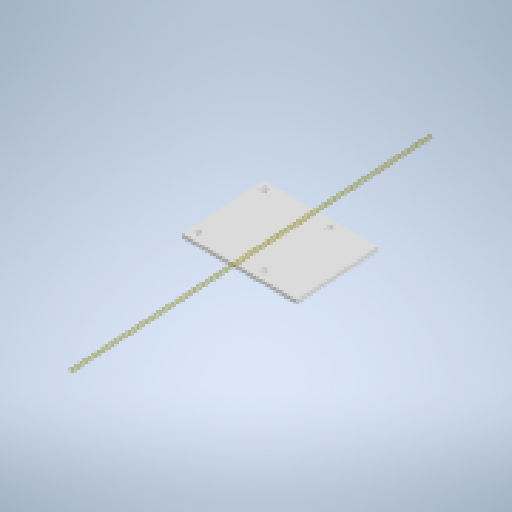
# Autodesk Inventor part: X axis carriage
Saved by Autodesk Inventor 2023.2 (Build 272271000, 271)
## iProperties
Created: 2023-05-09
Part Number: X axis carriage
Material: Generic
Document SubType Name: Modeling
Designer: dmargari
Density: 1 g/cm^3
Appearance: Default
Author: dmargari
Autodesk Inventor part; units mm, degrees
ref_plane "YZ Plane" through (0, 0, 0) normal (1, 0, 0) x (0, 1, 0)
ref_plane "XZ Plane" through (0, 0, 0) normal (0, 1, 0) x (-1, 0, 0)
ref_plane "XY Plane" through (0, 0, 0) normal (0, 0, 1) x (1, 0, 0)
ref_plane "Work Plane1" through (-11.5353, 732.2171, -211.5196) normal (-0.0000012, -0.9978756, -0.0651475) x (1, -0.0000012, -0.0000001)
sketch "Sketch2" plane through (-11.5353, 732.2171, -211.5196) normal (-0.0000012, -0.9978756, -0.0651475) x (1, -0.0000012, -0.0000001)
  line L0 (47.2205, 275.3712) -> (-77.9795, 275.3712)
  line L1 (-77.9795, 275.3712) -> (-77.9795, 150.1712)
  line L2 (-77.9795, 150.1712) -> (47.2205, 150.1712)
  line L3 (47.2205, 150.1712) -> (47.2205, 275.3712) construction
  line L4 (47.2205, 275.3712) -> (97.2205, 275.3712)
  line L5 (97.2205, 275.3712) -> (97.2205, 150.1712)
  line L6 (97.2205, 150.1712) -> (47.2205, 150.1712)
  line L7 (34.9205, 141.5153) -> (34.9205, 309.2543) construction
  line L8 (-65.6795, 309.2543) -> (-65.6795, 110.7061) construction
  line L9 (72.2205, 263.0712) -> (-113.8811, 263.0712) construction
  line L10 (72.2205, 162.4712) -> (-118.8511, 162.4712) construction
  point P0 (11.5362, 258.7723)
  point P1 (-138.0714, 537.573)
  point P2 (-211.9698, 678.1667)
  point P3 (34.9205, 263.0712)
  point P4 (34.9205, 162.4712)
  point P5 (-65.6795, 162.4712)
  point P6 (-65.6795, 263.0712)
  dimension "d15" = 125.2
  dimension "d16" = 125.2
  dimension "d23" = 50
  dimension "d30" = 12.3
  dimension "d31" = 100.6
  dimension "d32" = 12.3
  dimension "d33" = 100.6
  constraints: 22 end point, 9 point on line, 4 perpendicular, 3 horizontal, 2 parallel, 1 collinear, 1 vertical
  measures "d15" distance of L2.end L1.end
  measures "d16" distance of L1.end L0.end
  measures "d23" distance of L0.start L4.end
  measures "d30" distance between parallel lines of L0 L9
  measures "d31" distance between parallel lines of L9 L10
  measures "d32" distance between parallel lines of L3 L7
  measures "d33" distance between parallel lines of L7 L8
extrude "Extrusion2" add sketch "Sketch2" along normal blind 6
hole "Hole1" at (23.3852, 715.0787, 50.9927) at (23.3852, 721.6325, -49.3936) at (-77.2148, 715.0788, 50.9927) direction (-0.0000012, -0.9978756, -0.0651475) diameter 5.1 end through all counterbore diameter 9.2 counterbore depth 2
hole "Hole2" at (-77.2148, 721.6326, -49.3935) direction (-0.0000012, -0.9978756, -0.0651475) diameter 7.2 end through all counterbore diameter 12.25 counterbore depth 2
body "Solid2"
